Autodesk Fusion 360 part; units mm, degrees
(part 3 of 12)
extrude "拉伸2" cut sketch "草图18" against normal blind 4 contours L4 L5 L6 L7 L8 L9 | L10 L11 L12 L13 L14 L15 | L16 L17 L18 L19 L20 L21 | L22 L23 L24 L25 L26 L27 | L28 L29 L30 L31 L32 L33 | L34 L35 L36 L37 L38 L39 | L40 L41 L42 L43 L44 L45 | L46 L47 L48 L49 L50 L51 | L52 L53 L54 L55 L56 L57 | L58 L59 L60 L61 L62 L63 | L64 L65 L66 L67 L68 L69 | L70 L71 L72 L73 L74 L75 | L76 L77 L78 L79 L80 L81 | L82 L83 L84 L85 L86 L87 | L88 L89 L90 L91 L92 L93 | L94 L95 L96 L97 L98 L99 | L100 L101 L102 L103 L104 L105 | L106 L107 L108 L109 L110 L111 | L112 L113 L114 L115 L116 L117 | L118 L119 L120 L121 L122 L123 | L124 L125 L126 L127 L128 L129 | L130 L131 L132 L133 L134 L135 | L136 L137 L138 L139 L140 L141 | L142 L143 L144 L145 L146 L147 | L148 L149 L150 L151 L152 L153 | L154 L155 L156 L157 L158 L159 | L160 L161 L162 L163 L164 L165 | L166 L167 L168 L169 L170 L171 | L172 L173 L174 L175 L176 L177 | L178 L179 L180 L181 L182 L183 | L184 L185 L186 L187 L188 L189 | L190 L191 L192 L193 L194 L195 | L196 L197 L198 L199 L200 L201 | L202 L203 L204 L205 L206 L207 | L208 L209 L210 L211 L212 L213 | L214 L215 L216 L217 L218 L219 | L220 L221 L222 L223 L224 L225 | L226 L227 L228 L229 L230 L231 | L232 L233 L234 L235 L236 L237 | L238 L239 L240 L241 L242 L243 | L244 L245 L246 L247 L248 L249 | L250 L251 L252 L253 L254 L255 | L256 L257 L258 L259 L260 L261 | L262 L263 L264 L265 L266 L267 | L268 L269 L270 L271 L272 L273 | L274 L275 L276 L277 L278 L279 | L280 L281 L282 L283 L284 L285 | L286 L287 L288 L289 L290 L291 | L292 L293 L294 L295 L296 L297 | L298 L299 L300 L301 L302 L303 | L304 L305 L306 L307 L308 L309 | L310 L311 L312 L313 L314 L315 | L316 L317 L318 L319 L320 L321 | L322 L323 L324 L325 L326 L327 | L328 L329 L330 L331 L332 L333 | L334 L335 L336 L337 L338 L339 | L340 L341 L342 L343 L344 L345 | L346 L347 L348 L349 L350 L351 | L352 L353 L354 L355 L356 L357 | L358 L359 L360 L361 L362 L363 | L364 L365 L366 L367 L368 L369 | L370 L371 L372 L373 L374 L375 | L376 L377 L378 L379 L380 L381 | L382 L383 L384 L385 L386 L387 | L388 L389 L390 L391 L392 L393 | L394 L395 L396 L397 L398 L399 | L400 L401 L402 L403 L404 L405 | L406 L407 L408 L409 L410 L411 | L412 L413 L414 L415 L416 L417 | L418 L419 L420 L421 L422 L423 | L424 L425 L426 L427 L428 L429 | L430 L431 L432 L433 L434 L435 | L436 L437 L438 L439 L440 L441 | L442 L443 L444 L445 L446 L447 | L448 L449 L450 L451 L452 L453 | L454 L455 L456 L457 L458 L459 | L460 L461 L462 L463 L464 L465 | L466 L467 L468 L469 L470 L471 | L472 L473 L474 L475 L476 L477 | L478 L479 L480 L481 L482 L483 | L484 L485 L486 L487 L488 L489 | L490 L491 L492 L493 L494 L495 | L496 L497 L498 L499 L500 L501 | L502 L503 L504 L505 L506 L507 | L508 L509 L510 L511 L512 L513 | L514 L515 L516 L517 L518 L519 | L520 L521 L522 L523 L524 L525 | L526 L527 L528 L529 L530 L531 | L532 L533 L534 L535 L536 L537 | L538 L539 L540 L541 L542 L543 | L544 L545 L546 L547 L548 L549 | L550 L551 L552 L553 L554 L555 | L556 L557 L558 L559 L560 L561 | L562 L563 L564 L565 L566 L567 | L568 L569 L570 L571 L572 L573 | L574 L575 L576 L577 L578 L579 | L580 L581 L582 L583 L584 L585 | L586 L587 L588 L589 L590 L591 | L592 L593 L594 L595 L596 L597 | L598 L599 L600 L601 L602 L603 | L604 L605 L606 L607 L608 L609 | L610 L611 L612 L613 L614 L615 | L616 L617 L618 L619 L620 L621 | L622 L623 L624 L625 L626 L627 | L628 L629 L630 L631 L632 L633 | L634 L635 L636 L637 L638 L639 | L640 L641 L642 L643 L644 L645 | L646 L647 L648 L649 L650 L651 | L652 L653 L654 L655 L656 L657 | L658 L659 L660 L661 L662 L663 | L664 L665 L666 L667 L668 L669 | L670 L671 L672 L673 L674 L675 | L676 L677 L678 L679 L680 L681 | L682 L683 L684 L685 L686 L687 | L688 L689 L690 L691 L692 L693 | L694 L695 L696 L697 L698 L699 | L700 L701 L702 L703 L704 L705 | L706 L707 L708 L709 L710 L711 | L712 L713 L714 L715 L716 L717 | L718 L719 L720 L721 L722 L723 | L724 L725 L726 L727 L728 L729 | L730 L731 L732 L733 L734 L735 | L736 L737 L738 L739 L740 L741 | L742 L743 L744 L745 L746 L747 | L748 L749 L750 L751 L752 L753 | L754 L755 L756 L757 L758 L759 | L760 L761 L762 L763 L764 L765 | L766 L767 L768 L769 L770 L771 | L772 L773 L774 L775 L776 L777 | L778 L779 L780 L781 L782 L783 | L784 L785 L786 L787 L788 L789 | L790 L791 L792 L793 L794 L795 | L796 L797 L798 L799 L800 L801 | L802 L803 L804 L805 L806 L807 | L808 L809 L810 L811 L812 L813 | L814 L815 L816 L817 L818 L819 | L820 L821 L822 L823 L824 L825 | L826 L827 L828 L829 L830 L831 | L832 L833 L834 L835 L836 L837 | L838 L839 L840 L841 L842 L843 | L844 L845 L846 L847 L848 L849 | L850 L851 L852 L853 L854 L855 | L856 L857 L858 L859 L860 L861 | L862 L863 L864 L865 L866 L867 | L868 L869 L870 L871 L872 L873 | L874 L875 L876 L877 L878 L879 | L880 L881 L882 L883 L884 L885 | L886 L887 L888 L889 L890 L891 | L892 L893 L894 L895 L896 L897 | L898 L899 L900 L901 L902 L903 | L904 L905 L906 L907 L908 L909 | L910 L911 L912 L913 L914 L915 | L916 L917 L918 L919 L920 L921 | L922 L923 L924 L925 L926 L927 | L928 L929 L930 L931 L932 L933 | L934 L935 L936 L937 L938 L939 | L940 L941 L942 L943 L944 L945 | L946 L947 L948 L949 L950 L951 | L952 L953 L954 L955 L956 L957 | L958 L959 L960 L961 L962 L963 | L964 L965 L966 L967 L968 L969 | L970 L971 L972 L973 L974 L975 | L976 L977 L978 L979 L980 L981 | L982 L983 L984 L985 L986 L987 | L988 L989 L990 L991 L992 L993 | L994 L995 L996 L997 L998 L999 | L1000 L1001 L1002 L1003 L1004 L1005 | L1006 L1007 L1008 L1009 L1010 L1011 | L1012 L1013 L1014 L1015 L1016 L1017 | L1018 L1019 L1020 L1021 L1022 L1023 | L1024 L1025 L1026 L1027 L1028 L1029 | L1030 L1031 L1032 L1033 L1034 L1035 | L1036 L1037 L1038 L1039 L1040 L1041 | L1042 L1043 L1044 L1045 L1046 L1047 | L1048 L1049 L1050 L1051 L1052 L1053 | L1054 L1055 L1056 L1057 L1058 L1059 | L1060 L1061 L1062 L1063 L1064 L1065 | L1066 L1067 L1068 L1069 L1070 L1071 | L1072 L1073 L1074 L1075 L1076 L1077 | L1078 L1079 L1080 L1081 L1082 L1083 | L1084 L1085 L1086 L1087 L1088 L1089 | L1090 L1091 L1092 L1093 L1094 L1095 | L1096 L1097 L1098 L1099 L1100 L1101 | L1102 L1103 L1104 L1105 L1106 L1107 | L1108 L1109 L1110 L1111 L1112 L1113 | L1114 L1115 L1116 L1117 L1118 L1119 | L1120 L1121 L1122 L1123 L1124 L1125 | L1126 L1127 L1128 L1129 L1130 L1131 | L1132 L1133 L1134 L1135 L1136 L1137 | L1138 L1139 L1140 L1141 L1142 L1143 | L1144 L1145 L1146 L1147 L1148 L1149 | L1150 L1151 L1152 L1153 L1154 L1155 | L1156 L1157 L1158 L1159 L1160 L1161 | L1162 L1163 L1164 L1165 L1166 L1167 | L1168 L1169 L1170 L1171 L1172 L1173 | L1174 L1175 L1176 L1177 L1178 L1179 | L1180 L1181 L1182 L1183 L1184 L1185 | L1186 L1187 L1188 L1189 L1190 L1191 | L1192 L1193 L1194 L1195 L1196 L1197 | L1198 L1199 L1200 L1201 L1202 L1203 | L1204 L1205 L1206 L1207 L1208 L1209 | L1210 L1211 L1212 L1213 L1214 L1215 | L1216 L1217 L1218 L1219 L1220 L1221 | L1222 L1223 L1224 L1225 L1226 L1227 | L1228 L1229 L1230 L1231 L1232 L1233 | L1234 L1235 L1236 L1237 L1238 L1239 | L1240 L1241 L1242 L1243 L1244 L1245 | L1246 L1247 L1248 L1249 L1250 L1251 | L1252 L1253 L1254 L1255 L1256 L1257 | L1258 L1259 L1260 L1261 L1262 L1263 | L1264 L1265 L1266 L1267 L1268 L1269 | L1270 L1271 L1272 L1273 L1274 L1275 | L1276 L1277 L1278 L1279 L1280 L1281 | L1282 L1283 L1284 L1285 L1286 L1287 | L1288 L1289 L1290 L1291 L1292 L1293 | L1294 L1295 L1296 L1297 L1298 L1299 | L1300 L1301 L1302 L1303 L1304 L1305 | L1306 L1307 L1308 L1309 L1310 L1311 | L1312 L1313 L1314 L1315 L1316 L1317 | L1318 L1319 L1320 L1321 L1322 L1323 | L1324 L1325 L1326 L1327 L1328 L1329 | L1330 L1331 L1332 L1333 L1334 L1335 | L1336 L1337 L1338 L1339 L1340 L1341 | L1342 L1343 L1344 L1345 L1346 L1347 | L1348 L1349 L1350 L1351 L1352 L1353 | L1354 L1355 L1356 L1357 L1358 L1359 | L1360 L1361 L1362 L1363 L1364 L1365 | L1366 L1367 L1368 L1369 L1370 L1371 | L1372 L1373 L1374 L1375 L1376 L1377 | L1378 L1379 L1380 L1381 L1382 L1383 | L1384 L1385 L1386 L1387 L1388 L1389 | L1390 L1391 L1392 L1393 L1394 L1395 | L1396 L1397 L1398 L1399 L1400 L1401 | L1402 L1403 L1404 L1405 L1406 L1407 | L1408 L1409 L1410 L1411 L1412 L1413 | L1414 L1415 L1416 L1417 L1418 L1419 | L1420 L1421 L1422 L1423 L1424 L1425 | L1426 L1427 L1428 L1429 L1430 L1431 | L1432 L1433 L1434 L1435 L1436 L1437 | L1438 L1439 L1440 L1441 L1442 L1443 | L1444 L1445 L1446 L1447 L1448 L1449 | L1450 L1451 L1452 L1453 L1454 L1455 | L1456 L1457 L1458 L1459 L1460 L1461 | L1462 L1463 L1464 L1465 L1466 L1467 | L1468 L1469 L1470 L1471 L1472 L1473 | L1474 L1475 L1476 L1477 L1478 L1479 | L1480 L1481 L1482 L1483 L1484 L1485 | L1486 L1487 L1488 L1489 L1490 L1491 | L1492 L1493 L1494 L1495 L1496 L1497 | L1498 L1499 L1500 L1501 L1502 L1503 | L1504 L1505 L1506 L1507 L1508 L1509 | L1510 L1511 L1512 L1513 L1514 L1515 | L1516 L1517 L1518 L1519 L1520 L1521 | L1522 L1523 L1524 L1525 L1526 L1527 | L1528 L1529 L1530 L1531 L1532 L1533 | L1534 L1535 L1536 L1537 L1538 L1539 | L1540 L1541 L1542 L1543 L1544 L1545 | L1546 L1547 L1548 L1549 L1550 L1551 | L1552 L1553 L1554 L1555 L1556 L1557 | L1558 L1559 L1560 L1561 L1562 L1563 | L1564 L1565 L1566 L1567 L1568 L1569 | L1570 L1571 L1572 L1573 L1574 L1575 | L1576 L1577 L1578 L1579 L1580 L1581 | L1582 L1583 L1584 L1585 L1586 L1587 | L1588 L1589 L1590 L1591 L1592 L1593 | L1594 L1595 L1596 L1597 L1598 L1599 | L1600 L1601 L1602 L1603 L1604 L1605 | L1606 L1607 L1608 L1609 L1610 L1611 | L1612 L1613 L1614 L1615 L1616 L1617 | L1618 L1619 L1620 L1621 L1622 L1623 | L1624 L1625 L1626 L1627 L1628 L1629 | L1630 L1631 L1632 L1633 L1634 L1635 | L1636 L1637 L1638 L1639 L1640 L1641 | L1642 L1643 L1644 L1645 L1646 L1647 | L1648 L1649 L1650 L1651 L1652 L1653
sketch "草图26" plane through (0, 73.5, 0) normal (0, -1, 0) x (1, 0, 0)
  line L0 (-60, 0) -> (60, 0)
  line L1 (60, 0) -> (60, 250)
  line L2 (60, 250) -> (-60, 250)
  line L3 (-60, 250) -> (-60, 0)
  line L4 (-50, 15) -> (-54.3301, 12.5)
  line L5 (-54.3301, 12.5) -> (-54.3301, 7.5)
  line L6 (-54.3301, 7.5) -> (-50, 5)
  line L7 (-50, 5) -> (-45.6699, 7.5)
  line L8 (-45.6699, 7.5) -> (-45.6699, 12.5)
  line L9 (-45.6699, 12.5) -> (-50, 15)
  line L10 (-39.3397, 15) -> (-43.6699, 12.5)
  line L11 (-43.6699, 12.5) -> (-43.6699, 7.5)
  line L12 (-43.6699, 7.5) -> (-39.3397, 5)
  line L13 (-39.3397, 5) -> (-35.0096, 7.5)
  line L14 (-35.0096, 7.5) -> (-35.0096, 12.5)
  line L15 (-35.0096, 12.5) -> (-39.3397, 15)
  line L16 (-28.6795, 15) -> (-33.0096, 12.5)
  line L17 (-33.0096, 12.5) -> (-33.0096, 7.5)
  line L18 (-33.0096, 7.5) -> (-28.6795, 5)
  line L19 (-28.6795, 5) -> (-24.3494, 7.5)
  line L20 (-24.3494, 7.5) -> (-24.3494, 12.5)
  line L21 (-24.3494, 12.5) -> (-28.6795, 15)
  line L22 (-18.0192, 15) -> (-22.3494, 12.5)
  line L23 (-22.3494, 12.5) -> (-22.3494, 7.5)
  line L24 (-22.3494, 7.5) -> (-18.0192, 5)
  line L25 (-18.0192, 5) -> (-13.6891, 7.5)
  line L26 (-13.6891, 7.5) -> (-13.6891, 12.5)
  line L27 (-13.6891, 12.5) -> (-18.0192, 15)
  line L28 (-7.359, 15) -> (-11.6891, 12.5)
  line L29 (-11.6891, 12.5) -> (-11.6891, 7.5)
  line L30 (-11.6891, 7.5) -> (-7.359, 5)
  line L31 (-7.359, 5) -> (-3.0289, 7.5)
  line L32 (-3.0289, 7.5) -> (-3.0289, 12.5)
  line L33 (-3.0289, 12.5) -> (-7.359, 15)
  line L34 (3.3013, 15) -> (-1.0289, 12.5)
  line L35 (-1.0289, 12.5) -> (-1.0289, 7.5)
  line L36 (-1.0289, 7.5) -> (3.3013, 5)
  line L37 (3.3013, 5) -> (7.6314, 7.5)
  line L38 (7.6314, 7.5) -> (7.6314, 12.5)
  line L39 (7.6314, 12.5) -> (3.3013, 15)
  line L40 (13.9615, 15) -> (9.6314, 12.5)
  line L41 (9.6314, 12.5) -> (9.6314, 7.5)
  line L42 (9.6314, 7.5) -> (13.9615, 5)
  line L43 (13.9615, 5) -> (18.2917, 7.5)
  line L44 (18.2917, 7.5) -> (18.2917, 12.5)
  line L45 (18.2917, 12.5) -> (13.9615, 15)
  line L46 (24.6218, 15) -> (20.2917, 12.5)
  line L47 (20.2917, 12.5) -> (20.2917, 7.5)
  line L48 (20.2917, 7.5) -> (24.6218, 5)
  line L49 (24.6218, 5) -> (28.9519, 7.5)
  line L50 (28.9519, 7.5) -> (28.9519, 12.5)
  line L51 (28.9519, 12.5) -> (24.6218, 15)
  line L52 (35.282, 15) -> (30.9519, 12.5)
  line L53 (30.9519, 12.5) -> (30.9519, 7.5)
  line L54 (30.9519, 7.5) -> (35.282, 5)
  line L55 (35.282, 5) -> (39.6122, 7.5)
  line L56 (39.6122, 7.5) -> (39.6122, 12.5)
  line L57 (39.6122, 12.5) -> (35.282, 15)
  line L58 (45.9423, 15) -> (41.6122, 12.5)
  line L59 (41.6122, 12.5) -> (41.6122, 7.5)
  line L60 (41.6122, 7.5) -> (45.9423, 5)
  line L61 (45.9423, 5) -> (50.2724, 7.5)
  line L62 (50.2724, 7.5) -> (50.2724, 12.5)
  line L63 (50.2724, 12.5) -> (45.9423, 15)
  line L64 (-44.6699, 24.2321) -> (-49, 21.7321)
  line L65 (-49, 21.7321) -> (-49, 16.7321)
  line L66 (-49, 16.7321) -> (-44.6699, 14.2321)
  line L67 (-44.6699, 14.2321) -> (-40.3397, 16.7321)
  line L68 (-40.3397, 16.7321) -> (-40.3397, 21.7321)
  line L69 (-40.3397, 21.7321) -> (-44.6699, 24.2321)
  line L70 (-34.0096, 24.2321) -> (-38.3397, 21.7321)
  line L71 (-38.3397, 21.7321) -> (-38.3397, 16.7321)
  line L72 (-38.3397, 16.7321) -> (-34.0096, 14.2321)
  line L73 (-34.0096, 14.2321) -> (-29.6795, 16.7321)
  line L74 (-29.6795, 16.7321) -> (-29.6795, 21.7321)
  line L75 (-29.6795, 21.7321) -> (-34.0096, 24.2321)
  line L76 (-23.3494, 24.2321) -> (-27.6795, 21.7321)
  line L77 (-27.6795, 21.7321) -> (-27.6795, 16.7321)
  line L78 (-27.6795, 16.7321) -> (-23.3494, 14.2321)
  line L79 (-23.3494, 14.2321) -> (-19.0192, 16.7321)
  line L80 (-19.0192, 16.7321) -> (-19.0192, 21.7321)
  line L81 (-19.0192, 21.7321) -> (-23.3494, 24.2321)
  line L82 (-12.6891, 24.2321) -> (-17.0192, 21.7321)
  line L83 (-17.0192, 21.7321) -> (-17.0192, 16.7321)
  line L84 (-17.0192, 16.7321) -> (-12.6891, 14.2321)
  line L85 (-12.6891, 14.2321) -> (-8.359, 16.7321)
  line L86 (-8.359, 16.7321) -> (-8.359, 21.7321)
  line L87 (-8.359, 21.7321) -> (-12.6891, 24.2321)
  line L88 (-2.0289, 24.2321) -> (-6.359, 21.7321)
  line L89 (-6.359, 21.7321) -> (-6.359, 16.7321)
  line L90 (-6.359, 16.7321) -> (-2.0289, 14.2321)
  line L91 (-2.0289, 14.2321) -> (2.3013, 16.7321)
  line L92 (2.3013, 16.7321) -> (2.3013, 21.7321)
  line L93 (2.3013, 21.7321) -> (-2.0289, 24.2321)
  line L94 (8.6314, 24.2321) -> (4.3013, 21.7321)
  line L95 (4.3013, 21.7321) -> (4.3013, 16.7321)
  line L96 (4.3013, 16.7321) -> (8.6314, 14.2321)
  line L97 (8.6314, 14.2321) -> (12.9615, 16.7321)
  line L98 (12.9615, 16.7321) -> (12.9615, 21.7321)
  line L99 (12.9615, 21.7321) -> (8.6314, 24.2321)
  line L100 (19.2917, 24.2321) -> (14.9615, 21.7321)
  line L101 (14.9615, 21.7321) -> (14.9615, 16.7321)
  line L102 (14.9615, 16.7321) -> (19.2917, 14.2321)
  line L103 (19.2917, 14.2321) -> (23.6218, 16.7321)
  line L104 (23.6218, 16.7321) -> (23.6218, 21.7321)
  line L105 (23.6218, 21.7321) -> (19.2917, 24.2321)
  line L106 (29.9519, 24.2321) -> (25.6218, 21.7321)
  line L107 (25.6218, 21.7321) -> (25.6218, 16.7321)
  line L108 (25.6218, 16.7321) -> (29.9519, 14.2321)
  line L109 (29.9519, 14.2321) -> (34.282, 16.7321)
  line L110 (34.282, 16.7321) -> (34.282, 21.7321)
  line L111 (34.282, 21.7321) -> (29.9519, 24.2321)
  line L112 (40.6122, 24.2321) -> (36.282, 21.7321)
  line L113 (36.282, 21.7321) -> (36.282, 16.7321)
  line L114 (36.282, 16.7321) -> (40.6122, 14.2321)
  line L115 (40.6122, 14.2321) -> (44.9423, 16.7321)
  line L116 (44.9423, 16.7321) -> (44.9423, 21.7321)
  line L117 (44.9423, 21.7321) -> (40.6122, 24.2321)
  line L118 (-50, 33.4641) -> (-54.3301, 30.9641)
  line L119 (-54.3301, 30.9641) -> (-54.3301, 25.9641)
  line L120 (-54.3301, 25.9641) -> (-50, 23.4641)
  line L121 (-50, 23.4641) -> (-45.6699, 25.9641)
  line L122 (-45.6699, 25.9641) -> (-45.6699, 30.9641)
  line L123 (-45.6699, 30.9641) -> (-50, 33.4641)
  line L124 (-39.3397, 33.4641) -> (-43.6699, 30.9641)
  line L125 (-43.6699, 30.9641) -> (-43.6699, 25.9641)
  line L126 (-43.6699, 25.9641) -> (-39.3397, 23.4641)
  line L127 (-39.3397, 23.4641) -> (-35.0096, 25.9641)
  line L128 (-35.0096, 25.9641) -> (-35.0096, 30.9641)
  line L129 (-35.0096, 30.9641) -> (-39.3397, 33.4641)
  line L130 (-28.6795, 33.4641) -> (-33.0096, 30.9641)
  line L131 (-33.0096, 30.9641) -> (-33.0096, 25.9641)
  line L132 (-33.0096, 25.9641) -> (-28.6795, 23.4641)
  line L133 (-28.6795, 23.4641) -> (-24.3494, 25.9641)
  line L134 (-24.3494, 25.9641) -> (-24.3494, 30.9641)
  line L135 (-24.3494, 30.9641) -> (-28.6795, 33.4641)
  line L136 (-18.0192, 33.4641) -> (-22.3494, 30.9641)
  line L137 (-22.3494, 30.9641) -> (-22.3494, 25.9641)
  line L138 (-22.3494, 25.9641) -> (-18.0192, 23.4641)
  line L139 (-18.0192, 23.4641) -> (-13.6891, 25.9641)
  line L140 (-13.6891, 25.9641) -> (-13.6891, 30.9641)
  line L141 (-13.6891, 30.9641) -> (-18.0192, 33.4641)
  line L142 (-7.359, 33.4641) -> (-11.6891, 30.9641)
  line L143 (-11.6891, 30.9641) -> (-11.6891, 25.9641)
  line L144 (-11.6891, 25.9641) -> (-7.359, 23.4641)
  line L145 (-7.359, 23.4641) -> (-3.0289, 25.9641)
  line L146 (-3.0289, 25.9641) -> (-3.0289, 30.9641)
  line L147 (-3.0289, 30.9641) -> (-7.359, 33.4641)
  line L148 (3.3013, 33.4641) -> (-1.0289, 30.9641)
  line L149 (-1.0289, 30.9641) -> (-1.0289, 25.9641)
  line L150 (-1.0289, 25.9641) -> (3.3013, 23.4641)
  line L151 (3.3013, 23.4641) -> (7.6314, 25.9641)
  line L152 (7.6314, 25.9641) -> (7.6314, 30.9641)
  line L153 (7.6314, 30.9641) -> (3.3013, 33.4641)
  line L154 (13.9615, 33.4641) -> (9.6314, 30.9641)
  line L155 (9.6314, 30.9641) -> (9.6314, 25.9641)
  line L156 (9.6314, 25.9641) -> (13.9615, 23.4641)
  line L157 (13.9615, 23.4641) -> (18.2917, 25.9641)
  line L158 (18.2917, 25.9641) -> (18.2917, 30.9641)
  line L159 (18.2917, 30.9641) -> (13.9615, 33.4641)
  line L160 (24.6218, 33.4641) -> (20.2917, 30.9641)
  line L161 (20.2917, 30.9641) -> (20.2917, 25.9641)
  line L162 (20.2917, 25.9641) -> (24.6218, 23.4641)
  line L163 (24.6218, 23.4641) -> (28.9519, 25.9641)
  line L164 (28.9519, 25.9641) -> (28.9519, 30.9641)
  line L165 (28.9519, 30.9641) -> (24.6218, 33.4641)
  line L166 (35.282, 33.4641) -> (30.9519, 30.9641)
  line L167 (30.9519, 30.9641) -> (30.9519, 25.9641)
  line L168 (30.9519, 25.9641) -> (35.282, 23.4641)
  line L169 (35.282, 23.4641) -> (39.6122, 25.9641)
  line L170 (39.6122, 25.9641) -> (39.6122, 30.9641)
  line L171 (39.6122, 30.9641) -> (35.282, 33.4641)
  line L172 (45.9423, 33.4641) -> (41.6122, 30.9641)
  line L173 (41.6122, 30.9641) -> (41.6122, 25.9641)
  line L174 (41.6122, 25.9641) -> (45.9423, 23.4641)
  line L175 (45.9423, 23.4641) -> (50.2724, 25.9641)
  line L176 (50.2724, 25.9641) -> (50.2724, 30.9641)
  line L177 (50.2724, 30.9641) -> (45.9423, 33.4641)
  line L178 (-44.6699, 42.6962) -> (-49, 40.1962)
  line L179 (-49, 40.1962) -> (-49, 35.1962)
  line L180 (-49, 35.1962) -> (-44.6699, 32.6962)
  line L181 (-44.6699, 32.6962) -> (-40.3397, 35.1962)
  line L182 (-40.3397, 35.1962) -> (-40.3397, 40.1962)
  line L183 (-40.3397, 40.1962) -> (-44.6699, 42.6962)
  line L184 (-34.0096, 42.6962) -> (-38.3397, 40.1962)
  line L185 (-38.3397, 40.1962) -> (-38.3397, 35.1962)
  line L186 (-38.3397, 35.1962) -> (-34.0096, 32.6962)
  line L187 (-34.0096, 32.6962) -> (-29.6795, 35.1962)
  line L188 (-29.6795, 35.1962) -> (-29.6795, 40.1962)
  line L189 (-29.6795, 40.1962) -> (-34.0096, 42.6962)
  line L190 (-23.3494, 42.6962) -> (-27.6795, 40.1962)
  line L191 (-27.6795, 40.1962) -> (-27.6795, 35.1962)
  line L192 (-27.6795, 35.1962) -> (-23.3494, 32.6962)
  line L193 (-23.3494, 32.6962) -> (-19.0192, 35.1962)
  line L194 (-19.0192, 35.1962) -> (-19.0192, 40.1962)
  line L195 (-19.0192, 40.1962) -> (-23.3494, 42.6962)
  line L196 (-12.6891, 42.6962) -> (-17.0192, 40.1962)
  line L197 (-17.0192, 40.1962) -> (-17.0192, 35.1962)
  line L198 (-17.0192, 35.1962) -> (-12.6891, 32.6962)
  line L199 (-12.6891, 32.6962) -> (-8.359, 35.1962)
  line L200 (-8.359, 35.1962) -> (-8.359, 40.1962)
  line L201 (-8.359, 40.1962) -> (-12.6891, 42.6962)
  line L202 (-2.0289, 42.6962) -> (-6.359, 40.1962)
  line L203 (-6.359, 40.1962) -> (-6.359, 35.1962)
  line L204 (-6.359, 35.1962) -> (-2.0289, 32.6962)
  line L205 (-2.0289, 32.6962) -> (2.3013, 35.1962)
  line L206 (2.3013, 35.1962) -> (2.3013, 40.1962)
  line L207 (2.3013, 40.1962) -> (-2.0289, 42.6962)
  line L208 (8.6314, 42.6962) -> (4.3013, 40.1962)
  line L209 (4.3013, 40.1962) -> (4.3013, 35.1962)
  line L210 (4.3013, 35.1962) -> (8.6314, 32.6962)
  line L211 (8.6314, 32.6962) -> (12.9615, 35.1962)
  line L212 (12.9615, 35.1962) -> (12.9615, 40.1962)
  line L213 (12.9615, 40.1962) -> (8.6314, 42.6962)
  line L214 (19.2917, 42.6962) -> (14.9615, 40.1962)
  line L215 (14.9615, 40.1962) -> (14.9615, 35.1962)
  line L216 (14.9615, 35.1962) -> (19.2917, 32.6962)
  line L217 (19.2917, 32.6962) -> (23.6218, 35.1962)
  line L218 (23.6218, 35.1962) -> (23.6218, 40.1962)
  line L219 (23.6218, 40.1962) -> (19.2917, 42.6962)
  line L220 (29.9519, 42.6962) -> (25.6218, 40.1962)
  line L221 (25.6218, 40.1962) -> (25.6218, 35.1962)
  line L222 (25.6218, 35.1962) -> (29.9519, 32.6962)
  line L223 (29.9519, 32.6962) -> (34.282, 35.1962)
  line L224 (34.282, 35.1962) -> (34.282, 40.1962)
  line L225 (34.282, 40.1962) -> (29.9519, 42.6962)
  line L226 (40.6122, 42.6962) -> (36.282, 40.1962)
  line L227 (36.282, 40.1962) -> (36.282, 35.1962)
  line L228 (36.282, 35.1962) -> (40.6122, 32.6962)
  line L229 (40.6122, 32.6962) -> (44.9423, 35.1962)
  line L230 (44.9423, 35.1962) -> (44.9423, 40.1962)
  line L231 (44.9423, 40.1962) -> (40.6122, 42.6962)
  line L232 (-50, 51.9282) -> (-54.3301, 49.4282)
  line L233 (-54.3301, 49.4282) -> (-54.3301, 44.4282)
  line L234 (-54.3301, 44.4282) -> (-50, 41.9282)
  line L235 (-50, 41.9282) -> (-45.6699, 44.4282)
  line L236 (-45.6699, 44.4282) -> (-45.6699, 49.4282)
  line L237 (-45.6699, 49.4282) -> (-50, 51.9282)
  line L238 (-39.3397, 51.9282) -> (-43.6699, 49.4282)
  line L239 (-43.6699, 49.4282) -> (-43.6699, 44.4282)
  line L240 (-43.6699, 44.4282) -> (-39.3397, 41.9282)
  line L241 (-39.3397, 41.9282) -> (-35.0096, 44.4282)
  line L242 (-35.0096, 44.4282) -> (-35.0096, 49.4282)
  line L243 (-35.0096, 49.4282) -> (-39.3397, 51.9282)
  line L244 (-28.6795, 51.9282) -> (-33.0096, 49.4282)
  line L245 (-33.0096, 49.4282) -> (-33.0096, 44.4282)
  line L246 (-33.0096, 44.4282) -> (-28.6795, 41.9282)
  line L247 (-28.6795, 41.9282) -> (-24.3494, 44.4282)
  line L248 (-24.3494, 44.4282) -> (-24.3494, 49.4282)
  line L249 (-24.3494, 49.4282) -> (-28.6795, 51.9282)
  line L250 (-18.0192, 51.9282) -> (-22.3494, 49.4282)
  line L251 (-22.3494, 49.4282) -> (-22.3494, 44.4282)
  line L252 (-22.3494, 44.4282) -> (-18.0192, 41.9282)
  line L253 (-18.0192, 41.9282) -> (-13.6891, 44.4282)
  line L254 (-13.6891, 44.4282) -> (-13.6891, 49.4282)
  line L255 (-13.6891, 49.4282) -> (-18.0192, 51.9282)
  line L256 (-7.359, 51.9282) -> (-11.6891, 49.4282)
  line L257 (-11.6891, 49.4282) -> (-11.6891, 44.4282)
  line L258 (-11.6891, 44.4282) -> (-7.359, 41.9282)
  line L259 (-7.359, 41.9282) -> (-3.0289, 44.4282)
  line L260 (-3.0289, 44.4282) -> (-3.0289, 49.4282)
  line L261 (-3.0289, 49.4282) -> (-7.359, 51.9282)
  line L262 (3.3013, 51.9282) -> (-1.0289, 49.4282)
  line L263 (-1.0289, 49.4282) -> (-1.0289, 44.4282)
  line L264 (-1.0289, 44.4282) -> (3.3013, 41.9282)
  line L265 (3.3013, 41.9282) -> (7.6314, 44.4282)
  line L266 (7.6314, 44.4282) -> (7.6314, 49.4282)
  line L267 (7.6314, 49.4282) -> (3.3013, 51.9282)
  line L268 (13.9615, 51.9282) -> (9.6314, 49.4282)
  line L269 (9.6314, 49.4282) -> (9.6314, 44.4282)
  line L270 (9.6314, 44.4282) -> (13.9615, 41.9282)
  line L271 (13.9615, 41.9282) -> (18.2917, 44.4282)
  line L272 (18.2917, 44.4282) -> (18.2917, 49.4282)
  line L273 (18.2917, 49.4282) -> (13.9615, 51.9282)
  line L274 (24.6218, 51.9282) -> (20.2917, 49.4282)
  line L275 (20.2917, 49.4282) -> (20.2917, 44.4282)
  line L276 (20.2917, 44.4282) -> (24.6218, 41.9282)
  line L277 (24.6218, 41.9282) -> (28.9519, 44.4282)
  line L278 (28.9519, 44.4282) -> (28.9519, 49.4282)
  line L279 (28.9519, 49.4282) -> (24.6218, 51.9282)
  line L280 (35.282, 51.9282) -> (30.9519, 49.4282)
  line L281 (30.9519, 49.4282) -> (30.9519, 44.4282)
  line L282 (30.9519, 44.4282) -> (35.282, 41.9282)
  line L283 (35.282, 41.9282) -> (39.6122, 44.4282)
  line L284 (39.6122, 44.4282) -> (39.6122, 49.4282)
  line L285 (39.6122, 49.4282) -> (35.282, 51.9282)
  line L286 (45.9423, 51.9282) -> (41.6122, 49.4282)
  line L287 (41.6122, 49.4282) -> (41.6122, 44.4282)
  line L288 (41.6122, 44.4282) -> (45.9423, 41.9282)
  line L289 (45.9423, 41.9282) -> (50.2724, 44.4282)
  line L290 (50.2724, 44.4282) -> (50.2724, 49.4282)
  line L291 (50.2724, 49.4282) -> (45.9423, 51.9282)
  line L292 (-44.6699, 61.1603) -> (-49, 58.6603)
  line L293 (-49, 58.6603) -> (-49, 53.6603)
  line L294 (-49, 53.6603) -> (-44.6699, 51.1603)
  line L295 (-44.6699, 51.1603) -> (-40.3397, 53.6603)
  line L296 (-40.3397, 53.6603) -> (-40.3397, 58.6603)
  line L297 (-40.3397, 58.6603) -> (-44.6699, 61.1603)
  line L298 (-34.0096, 61.1603) -> (-38.3397, 58.6603)
  line L299 (-38.3397, 58.6603) -> (-38.3397, 53.6603)
  line L300 (-38.3397, 53.6603) -> (-34.0096, 51.1603)
  line L301 (-34.0096, 51.1603) -> (-29.6795, 53.6603)
  line L302 (-29.6795, 53.6603) -> (-29.6795, 58.6603)
  line L303 (-29.6795, 58.6603) -> (-34.0096, 61.1603)
  line L304 (-23.3494, 61.1603) -> (-27.6795, 58.6603)
  line L305 (-27.6795, 58.6603) -> (-27.6795, 53.6603)
  line L306 (-27.6795, 53.6603) -> (-23.3494, 51.1603)
  line L307 (-23.3494, 51.1603) -> (-19.0192, 53.6603)
  line L308 (-19.0192, 53.6603) -> (-19.0192, 58.6603)
  line L309 (-19.0192, 58.6603) -> (-23.3494, 61.1603)
  line L310 (-12.6891, 61.1603) -> (-17.0192, 58.6603)
  line L311 (-17.0192, 58.6603) -> (-17.0192, 53.6603)
  line L312 (-17.0192, 53.6603) -> (-12.6891, 51.1603)
  line L313 (-12.6891, 51.1603) -> (-8.359, 53.6603)
  line L314 (-8.359, 53.6603) -> (-8.359, 58.6603)
  line L315 (-8.359, 58.6603) -> (-12.6891, 61.1603)
  line L316 (-2.0289, 61.1603) -> (-6.359, 58.6603)
  line L317 (-6.359, 58.6603) -> (-6.359, 53.6603)
  line L318 (-6.359, 53.6603) -> (-2.0289, 51.1603)
  line L319 (-2.0289, 51.1603) -> (2.3013, 53.6603)
  line L320 (2.3013, 53.6603) -> (2.3013, 58.6603)
  line L321 (2.3013, 58.6603) -> (-2.0289, 61.1603)
  line L322 (8.6314, 61.1603) -> (4.3013, 58.6603)
  line L323 (4.3013, 58.6603) -> (4.3013, 53.6603)
  line L324 (4.3013, 53.6603) -> (8.6314, 51.1603)
  line L325 (8.6314, 51.1603) -> (12.9615, 53.6603)
  line L326 (12.9615, 53.6603) -> (12.9615, 58.6603)
  line L327 (12.9615, 58.6603) -> (8.6314, 61.1603)
  line L328 (19.2917, 61.1603) -> (14.9615, 58.6603)
  line L329 (14.9615, 58.6603) -> (14.9615, 53.6603)
  line L330 (14.9615, 53.6603) -> (19.2917, 51.1603)
  line L331 (19.2917, 51.1603) -> (23.6218, 53.6603)
  line L332 (23.6218, 53.6603) -> (23.6218, 58.6603)
  line L333 (23.6218, 58.6603) -> (19.2917, 61.1603)
  line L334 (29.9519, 61.1603) -> (25.6218, 58.6603)
  line L335 (25.6218, 58.6603) -> (25.6218, 53.6603)
  line L336 (25.6218, 53.6603) -> (29.9519, 51.1603)
  line L337 (29.9519, 51.1603) -> (34.282, 53.6603)
  line L338 (34.282, 53.6603) -> (34.282, 58.6603)
  line L339 (34.282, 58.6603) -> (29.9519, 61.1603)
  line L340 (40.6122, 61.1603) -> (36.282, 58.6603)
  line L341 (36.282, 58.6603) -> (36.282, 53.6603)
  line L342 (36.282, 53.6603) -> (40.6122, 51.1603)
  line L343 (40.6122, 51.1603) -> (44.9423, 53.6603)
  line L344 (44.9423, 53.6603) -> (44.9423, 58.6603)
  line L345 (44.9423, 58.6603) -> (40.6122, 61.1603)
  line L346 (-50, 70.3923) -> (-54.3301, 67.8923)
  line L347 (-54.3301, 67.8923) -> (-54.3301, 62.8923)
  line L348 (-54.3301, 62.8923) -> (-50, 60.3923)
  line L349 (-50, 60.3923) -> (-45.6699, 62.8923)
  line L350 (-45.6699, 62.8923) -> (-45.6699, 67.8923)
  line L351 (-45.6699, 67.8923) -> (-50, 70.3923)
  line L352 (-39.3397, 70.3923) -> (-43.6699, 67.8923)
  line L353 (-43.6699, 67.8923) -> (-43.6699, 62.8923)
  line L354 (-43.6699, 62.8923) -> (-39.3397, 60.3923)
  line L355 (-39.3397, 60.3923) -> (-35.0096, 62.8923)
  line L356 (-35.0096, 62.8923) -> (-35.0096, 67.8923)
  line L357 (-35.0096, 67.8923) -> (-39.3397, 70.3923)
  line L358 (-28.6795, 70.3923) -> (-33.0096, 67.8923)
  line L359 (-33.0096, 67.8923) -> (-33.0096, 62.8923)
  line L360 (-33.0096, 62.8923) -> (-28.6795, 60.3923)
  line L361 (-28.6795, 60.3923) -> (-24.3494, 62.8923)
  line L362 (-24.3494, 62.8923) -> (-24.3494, 67.8923)
  line L363 (-24.3494, 67.8923) -> (-28.6795, 70.3923)
  line L364 (-18.0192, 70.3923) -> (-22.3494, 67.8923)
  line L365 (-22.3494, 67.8923) -> (-22.3494, 62.8923)
  line L366 (-22.3494, 62.8923) -> (-18.0192, 60.3923)
  line L367 (-18.0192, 60.3923) -> (-13.6891, 62.8923)
  line L368 (-13.6891, 62.8923) -> (-13.6891, 67.8923)
  line L369 (-13.6891, 67.8923) -> (-18.0192, 70.3923)
  line L370 (-7.359, 70.3923) -> (-11.6891, 67.8923)
  line L371 (-11.6891, 67.8923) -> (-11.6891, 62.8923)
  line L372 (-11.6891, 62.8923) -> (-7.359, 60.3923)
  line L373 (-7.359, 60.3923) -> (-3.0289, 62.8923)
  line L374 (-3.0289, 62.8923) -> (-3.0289, 67.8923)
  line L375 (-3.0289, 67.8923) -> (-7.359, 70.3923)
  line L376 (3.3013, 70.3923) -> (-1.0289, 67.8923)
  line L377 (-1.0289, 67.8923) -> (-1.0289, 62.8923)
  line L378 (-1.0289, 62.8923) -> (3.3013, 60.3923)
  line L379 (3.3013, 60.3923) -> (7.6314, 62.8923)
  line L380 (7.6314, 62.8923) -> (7.6314, 67.8923)
  line L381 (7.6314, 67.8923) -> (3.3013, 70.3923)
  line L382 (13.9615, 70.3923) -> (9.6314, 67.8923)
  line L383 (9.6314, 67.8923) -> (9.6314, 62.8923)
  line L384 (9.6314, 62.8923) -> (13.9615, 60.3923)
  line L385 (13.9615, 60.3923) -> (18.2917, 62.8923)
  line L386 (18.2917, 62.8923) -> (18.2917, 67.8923)
  line L387 (18.2917, 67.8923) -> (13.9615, 70.3923)
  line L388 (24.6218, 70.3923) -> (20.2917, 67.8923)
  line L389 (20.2917, 67.8923) -> (20.2917, 62.8923)
  line L390 (20.2917, 62.8923) -> (24.6218, 60.3923)
  line L391 (24.6218, 60.3923) -> (28.9519, 62.8923)
  line L392 (28.9519, 62.8923) -> (28.9519, 67.8923)
  line L393 (28.9519, 67.8923) -> (24.6218, 70.3923)
  line L394 (35.282, 70.3923) -> (30.9519, 67.8923)
  line L395 (30.9519, 67.8923) -> (30.9519, 62.8923)
  line L396 (30.9519, 62.8923) -> (35.282, 60.3923)
  line L397 (35.282, 60.3923) -> (39.6122, 62.8923)
  line L398 (39.6122, 62.8923) -> (39.6122, 67.8923)
  line L399 (39.6122, 67.8923) -> (35.282, 70.3923)
  line L400 (45.9423, 70.3923) -> (41.6122, 67.8923)
  line L401 (41.6122, 67.8923) -> (41.6122, 62.8923)
  line L402 (41.6122, 62.8923) -> (45.9423, 60.3923)
  line L403 (45.9423, 60.3923) -> (50.2724, 62.8923)
  line L404 (50.2724, 62.8923) -> (50.2724, 67.8923)
  line L405 (50.2724, 67.8923) -> (45.9423, 70.3923)
  line L406 (-44.6699, 79.6244) -> (-49, 77.1244)
  line L407 (-49, 77.1244) -> (-49, 72.1244)
  line L408 (-49, 72.1244) -> (-44.6699, 69.6244)
  line L409 (-44.6699, 69.6244) -> (-40.3397, 72.1244)
  line L410 (-40.3397, 72.1244) -> (-40.3397, 77.1244)
  line L411 (-40.3397, 77.1244) -> (-44.6699, 79.6244)
  line L412 (-34.0096, 79.6244) -> (-38.3397, 77.1244)
  line L413 (-38.3397, 77.1244) -> (-38.3397, 72.1244)
  line L414 (-38.3397, 72.1244) -> (-34.0096, 69.6244)
  line L415 (-34.0096, 69.6244) -> (-29.6795, 72.1244)
  line L416 (-29.6795, 72.1244) -> (-29.6795, 77.1244)
  line L417 (-29.6795, 77.1244) -> (-34.0096, 79.6244)
  line L418 (-23.3494, 79.6244) -> (-27.6795, 77.1244)
  line L419 (-27.6795, 77.1244) -> (-27.6795, 72.1244)
  line L420 (-27.6795, 72.1244) -> (-23.3494, 69.6244)
  line L421 (-23.3494, 69.6244) -> (-19.0192, 72.1244)
  line L422 (-19.0192, 72.1244) -> (-19.0192, 77.1244)
  line L423 (-19.0192, 77.1244) -> (-23.3494, 79.6244)
  line L424 (-12.6891, 79.6244) -> (-17.0192, 77.1244)
  line L425 (-17.0192, 77.1244) -> (-17.0192, 72.1244)
  line L426 (-17.0192, 72.1244) -> (-12.6891, 69.6244)
  line L427 (-12.6891, 69.6244) -> (-8.359, 72.1244)
  line L428 (-8.359, 72.1244) -> (-8.359, 77.1244)
  line L429 (-8.359, 77.1244) -> (-12.6891, 79.6244)
  line L430 (-2.0289, 79.6244) -> (-6.359, 77.1244)
  line L431 (-6.359, 77.1244) -> (-6.359, 72.1244)
  line L432 (-6.359, 72.1244) -> (-2.0289, 69.6244)
  line L433 (-2.0289, 69.6244) -> (2.3013, 72.1244)
  line L434 (2.3013, 72.1244) -> (2.3013, 77.1244)
  line L435 (2.3013, 77.1244) -> (-2.0289, 79.6244)
  line L436 (8.6314, 79.6244) -> (4.3013, 77.1244)
  line L437 (4.3013, 77.1244) -> (4.3013, 72.1244)
  line L438 (4.3013, 72.1244) -> (8.6314, 69.6244)
  line L439 (8.6314, 69.6244) -> (12.9615, 72.1244)
  line L440 (12.9615, 72.1244) -> (12.9615, 77.1244)
  line L441 (12.9615, 77.1244) -> (8.6314, 79.6244)
  line L442 (19.2917, 79.6244) -> (14.9615, 77.1244)
  line L443 (14.9615, 77.1244) -> (14.9615, 72.1244)
  line L444 (14.9615, 72.1244) -> (19.2917, 69.6244)
  line L445 (19.2917, 69.6244) -> (23.6218, 72.1244)
  line L446 (23.6218, 72.1244) -> (23.6218, 77.1244)
  line L447 (23.6218, 77.1244) -> (19.2917, 79.6244)
  line L448 (29.9519, 79.6244) -> (25.6218, 77.1244)
  line L449 (25.6218, 77.1244) -> (25.6218, 72.1244)
  line L450 (25.6218, 72.1244) -> (29.9519, 69.6244)
  line L451 (29.9519, 69.6244) -> (34.282, 72.1244)
  line L452 (34.282, 72.1244) -> (34.282, 77.1244)
  line L453 (34.282, 77.1244) -> (29.9519, 79.6244)
  line L454 (40.6122, 79.6244) -> (36.282, 77.1244)
  line L455 (36.282, 77.1244) -> (36.282, 72.1244)
  line L456 (36.282, 72.1244) -> (40.6122, 69.6244)
  line L457 (40.6122, 69.6244) -> (44.9423, 72.1244)
  line L458 (44.9423, 72.1244) -> (44.9423, 77.1244)
  line L459 (44.9423, 77.1244) -> (40.6122, 79.6244)
  line L460 (-50, 88.8564) -> (-54.3301, 86.3564)
  line L461 (-54.3301, 86.3564) -> (-54.3301, 81.3564)
  line L462 (-54.3301, 81.3564) -> (-50, 78.8564)
  line L463 (-50, 78.8564) -> (-45.6699, 81.3564)
  line L464 (-45.6699, 81.3564) -> (-45.6699, 86.3564)
  line L465 (-45.6699, 86.3564) -> (-50, 88.8564)
  line L466 (-39.3397, 88.8564) -> (-43.6699, 86.3564)
  line L467 (-43.6699, 86.3564) -> (-43.6699, 81.3564)
  line L468 (-43.6699, 81.3564) -> (-39.3397, 78.8564)
  line L469 (-39.3397, 78.8564) -> (-35.0096, 81.3564)
  line L470 (-35.0096, 81.3564) -> (-35.0096, 86.3564)
  line L471 (-35.0096, 86.3564) -> (-39.3397, 88.8564)
  line L472 (-28.6795, 88.8564) -> (-33.0096, 86.3564)
  line L473 (-33.0096, 86.3564) -> (-33.0096, 81.3564)
  line L474 (-33.0096, 81.3564) -> (-28.6795, 78.8564)
  line L475 (-28.6795, 78.8564) -> (-24.3494, 81.3564)
  line L476 (-24.3494, 81.3564) -> (-24.3494, 86.3564)
  line L477 (-24.3494, 86.3564) -> (-28.6795, 88.8564)
  line L478 (-18.0192, 88.8564) -> (-22.3494, 86.3564)
  line L479 (-22.3494, 86.3564) -> (-22.3494, 81.3564)
  line L480 (-22.3494, 81.3564) -> (-18.0192, 78.8564)
  line L481 (-18.0192, 78.8564) -> (-13.6891, 81.3564)
  line L482 (-13.6891, 81.3564) -> (-13.6891, 86.3564)
  line L483 (-13.6891, 86.3564) -> (-18.0192, 88.8564)
  line L484 (-7.359, 88.8564) -> (-11.6891, 86.3564)
  line L485 (-11.6891, 86.3564) -> (-11.6891, 81.3564)
  line L486 (-11.6891, 81.3564) -> (-7.359, 78.8564)
  line L487 (-7.359, 78.8564) -> (-3.0289, 81.3564)
  line L488 (-3.0289, 81.3564) -> (-3.0289, 86.3564)
  line L489 (-3.0289, 86.3564) -> (-7.359, 88.8564)
  line L490 (3.3013, 88.8564) -> (-1.0289, 86.3564)
  line L491 (-1.0289, 86.3564) -> (-1.0289, 81.3564)
  line L492 (-1.0289, 81.3564) -> (3.3013, 78.8564)
  line L493 (3.3013, 78.8564) -> (7.6314, 81.3564)
  line L494 (7.6314, 81.3564) -> (7.6314, 86.3564)
  line L495 (7.6314, 86.3564) -> (3.3013, 88.8564)
  line L496 (13.9615, 88.8564) -> (9.6314, 86.3564)
  line L497 (9.6314, 86.3564) -> (9.6314, 81.3564)
  line L498 (9.6314, 81.3564) -> (13.9615, 78.8564)
  line L499 (13.9615, 78.8564) -> (18.2917, 81.3564)
  line L500 (18.2917, 81.3564) -> (18.2917, 86.3564)
  line L501 (18.2917, 86.3564) -> (13.9615, 88.8564)
  line L502 (24.6218, 88.8564) -> (20.2917, 86.3564)
  line L503 (20.2917, 86.3564) -> (20.2917, 81.3564)
  line L504 (20.2917, 81.3564) -> (24.6218, 78.8564)
  line L505 (24.6218, 78.8564) -> (28.9519, 81.3564)
  line L506 (28.9519, 81.3564) -> (28.9519, 86.3564)
  line L507 (28.9519, 86.3564) -> (24.6218, 88.8564)
  line L508 (35.282, 88.8564) -> (30.9519, 86.3564)
  line L509 (30.9519, 86.3564) -> (30.9519, 81.3564)
  line L510 (30.9519, 81.3564) -> (35.282, 78.8564)
  line L511 (35.282, 78.8564) -> (39.6122, 81.3564)
  line L512 (39.6122, 81.3564) -> (39.6122, 86.3564)
  line L513 (39.6122, 86.3564) -> (35.282, 88.8564)
  line L514 (45.9423, 88.8564) -> (41.6122, 86.3564)
  line L515 (41.6122, 86.3564) -> (41.6122, 81.3564)
  line L516 (41.6122, 81.3564) -> (45.9423, 78.8564)
  line L517 (45.9423, 78.8564) -> (50.2724, 81.3564)
  line L518 (50.2724, 81.3564) -> (50.2724, 86.3564)
  line L519 (50.2724, 86.3564) -> (45.9423, 88.8564)
  line L520 (-44.6699, 98.0885) -> (-49, 95.5885)
  line L521 (-49, 95.5885) -> (-49, 90.5885)
  line L522 (-49, 90.5885) -> (-44.6699, 88.0885)
  line L523 (-44.6699, 88.0885) -> (-40.3397, 90.5885)
  line L524 (-40.3397, 90.5885) -> (-40.3397, 95.5885)
  line L525 (-40.3397, 95.5885) -> (-44.6699, 98.0885)
  line L526 (-34.0096, 98.0885) -> (-38.3397, 95.5885)
  line L527 (-38.3397, 95.5885) -> (-38.3397, 90.5885)
  line L528 (-38.3397, 90.5885) -> (-34.0096, 88.0885)
  line L529 (-34.0096, 88.0885) -> (-29.6795, 90.5885)
  line L530 (-29.6795, 90.5885) -> (-29.6795, 95.5885)
  line L531 (-29.6795, 95.5885) -> (-34.0096, 98.0885)
  line L532 (-23.3494, 98.0885) -> (-27.6795, 95.5885)
  line L533 (-27.6795, 95.5885) -> (-27.6795, 90.5885)
  line L534 (-27.6795, 90.5885) -> (-23.3494, 88.0885)
  line L535 (-23.3494, 88.0885) -> (-19.0192, 90.5885)
  line L536 (-19.0192, 90.5885) -> (-19.0192, 95.5885)
  line L537 (-19.0192, 95.5885) -> (-23.3494, 98.0885)
  line L538 (-12.6891, 98.0885) -> (-17.0192, 95.5885)
  line L539 (-17.0192, 95.5885) -> (-17.0192, 90.5885)
  line L540 (-17.0192, 90.5885) -> (-12.6891, 88.0885)
  line L541 (-12.6891, 88.0885) -> (-8.359, 90.5885)
  line L542 (-8.359, 90.5885) -> (-8.359, 95.5885)
  line L543 (-8.359, 95.5885) -> (-12.6891, 98.0885)
  line L544 (-2.0289, 98.0885) -> (-6.359, 95.5885)
  line L545 (-6.359, 95.5885) -> (-6.359, 90.5885)
  line L546 (-6.359, 90.5885) -> (-2.0289, 88.0885)
  line L547 (-2.0289, 88.0885) -> (2.3013, 90.5885)
  line L548 (2.3013, 90.5885) -> (2.3013, 95.5885)
  line L549 (2.3013, 95.5885) -> (-2.0289, 98.0885)
  line L550 (8.6314, 98.0885) -> (4.3013, 95.5885)
  line L551 (4.3013, 95.5885) -> (4.3013, 90.5885)
  line L552 (4.3013, 90.5885) -> (8.6314, 88.0885)
  line L553 (8.6314, 88.0885) -> (12.9615, 90.5885)
  line L554 (12.9615, 90.5885) -> (12.9615, 95.5885)
  line L555 (12.9615, 95.5885) -> (8.6314, 98.0885)
  line L556 (19.2917, 98.0885) -> (14.9615, 95.5885)
  line L557 (14.9615, 95.5885) -> (14.9615, 90.5885)
  line L558 (14.9615, 90.5885) -> (19.2917, 88.0885)
  line L559 (19.2917, 88.0885) -> (23.6218, 90.5885)
  line L560 (23.6218, 90.5885) -> (23.6218, 95.5885)
  line L561 (23.6218, 95.5885) -> (19.2917, 98.0885)
  line L562 (29.9519, 98.0885) -> (25.6218, 95.5885)
  line L563 (25.6218, 95.5885) -> (25.6218, 90.5885)
  line L564 (25.6218, 90.5885) -> (29.9519, 88.0885)
  line L565 (29.9519, 88.0885) -> (34.282, 90.5885)
  line L566 (34.282, 90.5885) -> (34.282, 95.5885)
  line L567 (34.282, 95.5885) -> (29.9519, 98.0885)
  line L568 (40.6122, 98.0885) -> (36.282, 95.5885)
  line L569 (36.282, 95.5885) -> (36.282, 90.5885)
  line L570 (36.282, 90.5885) -> (40.6122, 88.0885)
  line L571 (40.6122, 88.0885) -> (44.9423, 90.5885)
  line L572 (44.9423, 90.5885) -> (44.9423, 95.5885)
  line L573 (44.9423, 95.5885) -> (40.6122, 98.0885)
  line L574 (-50, 107.3205) -> (-54.3301, 104.8205)
  line L575 (-54.3301, 104.8205) -> (-54.3301, 99.8205)
  line L576 (-54.3301, 99.8205) -> (-50, 97.3205)
  line L577 (-50, 97.3205) -> (-45.6699, 99.8205)
  line L578 (-45.6699, 99.8205) -> (-45.6699, 104.8205)
  line L579 (-45.6699, 104.8205) -> (-50, 107.3205)
  line L580 (-39.3397, 107.3205) -> (-43.6699, 104.8205)
  line L581 (-43.6699, 104.8205) -> (-43.6699, 99.8205)
  line L582 (-43.6699, 99.8205) -> (-39.3397, 97.3205)
  line L583 (-39.3397, 97.3205) -> (-35.0096, 99.8205)
  line L584 (-35.0096, 99.8205) -> (-35.0096, 104.8205)
  line L585 (-35.0096, 104.8205) -> (-39.3397, 107.3205)
  line L586 (-28.6795, 107.3205) -> (-33.0096, 104.8205)
  line L587 (-33.0096, 104.8205) -> (-33.0096, 99.8205)
  line L588 (-33.0096, 99.8205) -> (-28.6795, 97.3205)
  line L589 (-28.6795, 97.3205) -> (-24.3494, 99.8205)
  line L590 (-24.3494, 99.8205) -> (-24.3494, 104.8205)
  line L591 (-24.3494, 104.8205) -> (-28.6795, 107.3205)
  line L592 (-18.0192, 107.3205) -> (-22.3494, 104.8205)
  line L593 (-22.3494, 104.8205) -> (-22.3494, 99.8205)
  line L594 (-22.3494, 99.8205) -> (-18.0192, 97.3205)
  line L595 (-18.0192, 97.3205) -> (-13.6891, 99.8205)
  line L596 (-13.6891, 99.8205) -> (-13.6891, 104.8205)
  line L597 (-13.6891, 104.8205) -> (-18.0192, 107.3205)
  line L598 (-7.359, 107.3205) -> (-11.6891, 104.8205)
  line L599 (-11.6891, 104.8205) -> (-11.6891, 99.8205)
  line L600 (-11.6891, 99.8205) -> (-7.359, 97.3205)
  line L601 (-7.359, 97.3205) -> (-3.0289, 99.8205)
  line L602 (-3.0289, 99.8205) -> (-3.0289, 104.8205)
  line L603 (-3.0289, 104.8205) -> (-7.359, 107.3205)
  line L604 (3.3013, 107.3205) -> (-1.0289, 104.8205)
  line L605 (-1.0289, 104.8205) -> (-1.0289, 99.8205)
  line L606 (-1.0289, 99.8205) -> (3.3013, 97.3205)
  line L607 (3.3013, 97.3205) -> (7.6314, 99.8205)
  line L608 (7.6314, 99.8205) -> (7.6314, 104.8205)
  line L609 (7.6314, 104.8205) -> (3.3013, 107.3205)
  line L610 (13.9615, 107.3205) -> (9.6314, 104.8205)
  line L611 (9.6314, 104.8205) -> (9.6314, 99.8205)
  line L612 (9.6314, 99.8205) -> (13.9615, 97.3205)
  line L613 (13.9615, 97.3205) -> (18.2917, 99.8205)
  line L614 (18.2917, 99.8205) -> (18.2917, 104.8205)
  line L615 (18.2917, 104.8205) -> (13.9615, 107.3205)
  line L616 (24.6218, 107.3205) -> (20.2917, 104.8205)
  line L617 (20.2917, 104.8205) -> (20.2917, 99.8205)
  line L618 (20.2917, 99.8205) -> (24.6218, 97.3205)
  line L619 (24.6218, 97.3205) -> (28.9519, 99.8205)
  line L620 (28.9519, 99.8205) -> (28.9519, 104.8205)
  line L621 (28.9519, 104.8205) -> (24.6218, 107.3205)
  line L622 (35.282, 107.3205) -> (30.9519, 104.8205)
  line L623 (30.9519, 104.8205) -> (30.9519, 99.8205)
  line L624 (30.9519, 99.8205) -> (35.282, 97.3205)
  line L625 (35.282, 97.3205) -> (39.6122, 99.8205)
  line L626 (39.6122, 99.8205) -> (39.6122, 104.8205)
  line L627 (39.6122, 104.8205) -> (35.282, 107.3205)
  line L628 (45.9423, 107.3205) -> (41.6122, 104.8205)
  line L629 (41.6122, 104.8205) -> (41.6122, 99.8205)
  line L630 (41.6122, 99.8205) -> (45.9423, 97.3205)
  line L631 (45.9423, 97.3205) -> (50.2724, 99.8205)
  line L632 (50.2724, 99.8205) -> (50.2724, 104.8205)
  line L633 (50.2724, 104.8205) -> (45.9423, 107.3205)
  line L634 (-44.6699, 116.5526) -> (-49, 114.0526)
  line L635 (-49, 114.0526) -> (-49, 109.0526)
  line L636 (-49, 109.0526) -> (-44.6699, 106.5526)
  line L637 (-44.6699, 106.5526) -> (-40.3397, 109.0526)
  line L638 (-40.3397, 109.0526) -> (-40.3397, 114.0526)
  line L639 (-40.3397, 114.0526) -> (-44.6699, 116.5526)
  line L640 (-34.0096, 116.5526) -> (-38.3397, 114.0526)
  line L641 (-38.3397, 114.0526) -> (-38.3397, 109.0526)
  line L642 (-38.3397, 109.0526) -> (-34.0096, 106.5526)
  line L643 (-34.0096, 106.5526) -> (-29.6795, 109.0526)
  line L644 (-29.6795, 109.0526) -> (-29.6795, 114.0526)
  line L645 (-29.6795, 114.0526) -> (-34.0096, 116.5526)
  line L646 (-23.3494, 116.5526) -> (-27.6795, 114.0526)
  line L647 (-27.6795, 114.0526) -> (-27.6795, 109.0526)
  line L648 (-27.6795, 109.0526) -> (-23.3494, 106.5526)
  line L649 (-23.3494, 106.5526) -> (-19.0192, 109.0526)
  line L650 (-19.0192, 109.0526) -> (-19.0192, 114.0526)
  line L651 (-19.0192, 114.0526) -> (-23.3494, 116.5526)
  line L652 (-12.6891, 116.5526) -> (-17.0192, 114.0526)
  line L653 (-17.0192, 114.0526) -> (-17.0192, 109.0526)
  line L654 (-17.0192, 109.0526) -> (-12.6891, 106.5526)
  line L655 (-12.6891, 106.5526) -> (-8.359, 109.0526)
  line L656 (-8.359, 109.0526) -> (-8.359, 114.0526)
  line L657 (-8.359, 114.0526) -> (-12.6891, 116.5526)
  line L658 (-2.0289, 116.5526) -> (-6.359, 114.0526)
  line L659 (-6.359, 114.0526) -> (-6.359, 109.0526)
  line L660 (-6.359, 109.0526) -> (-2.0289, 106.5526)
  line L661 (-2.0289, 106.5526) -> (2.3013, 109.0526)
  line L662 (2.3013, 109.0526) -> (2.3013, 114.0526)
  line L663 (2.3013, 114.0526) -> (-2.0289, 116.5526)
  line L664 (8.6314, 116.5526) -> (4.3013, 114.0526)
  line L665 (4.3013, 114.0526) -> (4.3013, 109.0526)
  line L666 (4.3013, 109.0526) -> (8.6314, 106.5526)
  line L667 (8.6314, 106.5526) -> (12.9615, 109.0526)
  line L668 (12.9615, 109.0526) -> (12.9615, 114.0526)
  line L669 (12.9615, 114.0526) -> (8.6314, 116.5526)
  line L670 (19.2917, 116.5526) -> (14.9615, 114.0526)
  line L671 (14.9615, 114.0526) -> (14.9615, 109.0526)
  line L672 (14.9615, 109.0526) -> (19.2917, 106.5526)
  line L673 (19.2917, 106.5526) -> (23.6218, 109.0526)
  line L674 (23.6218, 109.0526) -> (23.6218, 114.0526)
  line L675 (23.6218, 114.0526) -> (19.2917, 116.5526)
  line L676 (29.9519, 116.5526) -> (25.6218, 114.0526)
  line L677 (25.6218, 114.0526) -> (25.6218, 109.0526)
  line L678 (25.6218, 109.0526) -> (29.9519, 106.5526)
  line L679 (29.9519, 106.5526) -> (34.282, 109.0526)
  line L680 (34.282, 109.0526) -> (34.282, 114.0526)
  line L681 (34.282, 114.0526) -> (29.9519, 116.5526)
  line L682 (40.6122, 116.5526) -> (36.282, 114.0526)
  line L683 (36.282, 114.0526) -> (36.282, 109.0526)
  line L684 (36.282, 109.0526) -> (40.6122, 106.5526)
  line L685 (40.6122, 106.5526) -> (44.9423, 109.0526)
  line L686 (44.9423, 109.0526) -> (44.9423, 114.0526)
  line L687 (44.9423, 114.0526) -> (40.6122, 116.5526)
  line L688 (-50, 125.7846) -> (-54.3301, 123.2846)
  line L689 (-54.3301, 123.2846) -> (-54.3301, 118.2846)
  line L690 (-54.3301, 118.2846) -> (-50, 115.7846)
  line L691 (-50, 115.7846) -> (-45.6699, 118.2846)
  line L692 (-45.6699, 118.2846) -> (-45.6699, 123.2846)
  line L693 (-45.6699, 123.2846) -> (-50, 125.7846)
  line L694 (-39.3397, 125.7846) -> (-43.6699, 123.2846)
  line L695 (-43.6699, 123.2846) -> (-43.6699, 118.2846)
  line L696 (-43.6699, 118.2846) -> (-39.3397, 115.7846)
  line L697 (-39.3397, 115.7846) -> (-35.0096, 118.2846)
  line L698 (-35.0096, 118.2846) -> (-35.0096, 123.2846)
  line L699 (-35.0096, 123.2846) -> (-39.3397, 125.7846)
  line L700 (-28.6795, 125.7846) -> (-33.0096, 123.2846)
  line L701 (-33.0096, 123.2846) -> (-33.0096, 118.2846)
  line L702 (-33.0096, 118.2846) -> (-28.6795, 115.7846)
  line L703 (-28.6795, 115.7846) -> (-24.3494, 118.2846)
  line L704 (-24.3494, 118.2846) -> (-24.3494, 123.2846)
  line L705 (-24.3494, 123.2846) -> (-28.6795, 125.7846)
  line L706 (-18.0192, 125.7846) -> (-22.3494, 123.2846)
  line L707 (-22.3494, 123.2846) -> (-22.3494, 118.2846)
  line L708 (-22.3494, 118.2846) -> (-18.0192, 115.7846)
  line L709 (-18.0192, 115.7846) -> (-13.6891, 118.2846)
  line L710 (-13.6891, 118.2846) -> (-13.6891, 123.2846)
  line L711 (-13.6891, 123.2846) -> (-18.0192, 125.7846)
  line L712 (-7.359, 125.7846) -> (-11.6891, 123.2846)
  line L713 (-11.6891, 123.2846) -> (-11.6891, 118.2846)
  line L714 (-11.6891, 118.2846) -> (-7.359, 115.7846)
  line L715 (-7.359, 115.7846) -> (-3.0289, 118.2846)
  line L716 (-3.0289, 118.2846) -> (-3.0289, 123.2846)
  line L717 (-3.0289, 123.2846) -> (-7.359, 125.7846)
  line L718 (3.3013, 125.7846) -> (-1.0289, 123.2846)
  line L719 (-1.0289, 123.2846) -> (-1.0289, 118.2846)
  line L720 (-1.0289, 118.2846) -> (3.3013, 115.7846)
  line L721 (3.3013, 115.7846) -> (7.6314, 118.2846)
  line L722 (7.6314, 118.2846) -> (7.6314, 123.2846)
  line L723 (7.6314, 123.2846) -> (3.3013, 125.7846)
  line L724 (13.9615, 125.7846) -> (9.6314, 123.2846)
  line L725 (9.6314, 123.2846) -> (9.6314, 118.2846)
  line L726 (9.6314, 118.2846) -> (13.9615, 115.7846)
  line L727 (13.9615, 115.7846) -> (18.2917, 118.2846)
  line L728 (18.2917, 118.2846) -> (18.2917, 123.2846)
  line L729 (18.2917, 123.2846) -> (13.9615, 125.7846)
  line L730 (24.6218, 125.7846) -> (20.2917, 123.2846)
  line L731 (20.2917, 123.2846) -> (20.2917, 118.2846)
  line L732 (20.2917, 118.2846) -> (24.6218, 115.7846)
  line L733 (24.6218, 115.7846) -> (28.9519, 118.2846)
  line L734 (28.9519, 118.2846) -> (28.9519, 123.2846)
  line L735 (28.9519, 123.2846) -> (24.6218, 125.7846)
  line L736 (35.282, 125.7846) -> (30.9519, 123.2846)
  line L737 (30.9519, 123.2846) -> (30.9519, 118.2846)
  line L738 (30.9519, 118.2846) -> (35.282, 115.7846)
  line L739 (35.282, 115.7846) -> (39.6122, 118.2846)
  line L740 (39.6122, 118.2846) -> (39.6122, 123.2846)
  line L741 (39.6122, 123.2846) -> (35.282, 125.7846)
  line L742 (45.9423, 125.7846) -> (41.6122, 123.2846)
  line L743 (41.6122, 123.2846) -> (41.6122, 118.2846)
  line L744 (41.6122, 118.2846) -> (45.9423, 115.7846)
  line L745 (45.9423, 115.7846) -> (50.2724, 118.2846)
  line L746 (50.2724, 118.2846) -> (50.2724, 123.2846)
  line L747 (50.2724, 123.2846) -> (45.9423, 125.7846)
  line L748 (-44.6699, 135.0167) -> (-49, 132.5167)
  line L749 (-49, 132.5167) -> (-49, 127.5167)
  line L750 (-49, 127.5167) -> (-44.6699, 125.0167)
  line L751 (-44.6699, 125.0167) -> (-40.3397, 127.5167)
  line L752 (-40.3397, 127.5167) -> (-40.3397, 132.5167)
  line L753 (-40.3397, 132.5167) -> (-44.6699, 135.0167)
  line L754 (-34.0096, 135.0167) -> (-38.3397, 132.5167)
  line L755 (-38.3397, 132.5167) -> (-38.3397, 127.5167)
  line L756 (-38.3397, 127.5167) -> (-34.0096, 125.0167)
  line L757 (-34.0096, 125.0167) -> (-29.6795, 127.5167)
  line L758 (-29.6795, 127.5167) -> (-29.6795, 132.5167)
  line L759 (-29.6795, 132.5167) -> (-34.0096, 135.0167)
  line L760 (-23.3494, 135.0167) -> (-27.6795, 132.5167)
  line L761 (-27.6795, 132.5167) -> (-27.6795, 127.5167)
  line L762 (-27.6795, 127.5167) -> (-23.3494, 125.0167)
  line L763 (-23.3494, 125.0167) -> (-19.0192, 127.5167)
  line L764 (-19.0192, 127.5167) -> (-19.0192, 132.5167)
  line L765 (-19.0192, 132.5167) -> (-23.3494, 135.0167)
  line L766 (-12.6891, 135.0167) -> (-17.0192, 132.5167)
  line L767 (-17.0192, 132.5167) -> (-17.0192, 127.5167)